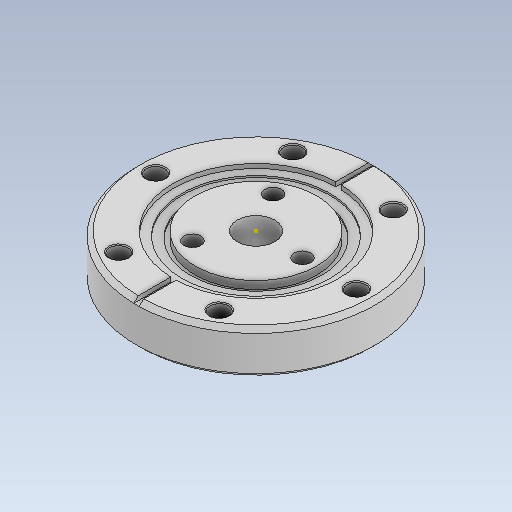
# Autodesk Inventor part: 2.75 flange
Saved by Autodesk Inventor 2020 (Build 240168000, 168)
## iProperties
Created: 2019-06-21
Part Number: 2.75 flange
Material: Generic
Document SubType Name: Modeling
Designer: ColinP
Density: 1 g/cm^3
Appearance: Default
Mass: 41.8424 g
Surface Area: 130.459 cm^2
Volume: 41.8424 cm^3
Author: ColinP
Autodesk Inventor part; units mm, degrees
ref_plane "YZ Plane" through (0, 0, 0) normal (1, 0, 0) x (0, 1, 0)
ref_plane "XZ Plane" through (0, 0, 0) normal (0, 1, 0) x (-1, 0, 0)
ref_plane "XY Plane" through (0, 0, 0) normal (0, 0, 1) x (1, 0, 0)
sketch "Sketch1" plane through (0, 0, 0) normal (0, 1, 0) x (-1, 0, 0)
  circle A0 centre (0, 0) radius 34.925
  dimension "d0" = 69.85
  constraints: 1 centre point, 1 coincident
  measures "d0" diameter of A0
extrude "Extrusion1" add sketch "Sketch1" along normal blind 12.7
sketch "Sketch2" plane through (0, 12.7, 0) normal (0, 1, 0) x (1, 0, 0)
  circle A0 centre (0, 0) radius 17.78
  circle A1 centre (0, 0) radius 19.05
  circle A2 centre (0, 0) radius 21.59
  circle A3 centre (0, 0) radius 24.13
  dimension "d3" = 35.56
  dimension "d4" = 38.1
  dimension "d5" = 43.18
  dimension "d6" = 48.26
  constraints: 4 centre point, 4 coincident
  measures "d3" diameter of A0
  measures "d4" diameter of A1
  measures "d5" diameter of A2
  measures "d6" diameter of A3
extrude "Extrusion2" cut sketch "Sketch2" against normal blind 1.27 contours A3
extrude "Extrusion3" cut sketch "Sketch2" against normal blind 1.778 contours A2
extrude "Extrusion4" cut sketch "Sketch2" against normal blind 2.286 contours A1
sketch "Sketch3" plane through (0, 0, 0) normal (0, -1, 0) x (1, 0, 0)
  circle A0 centre (0, 0) radius 19.05
  circle A1 centre (0, 0) radius 21.59
  circle A2 centre (0, 0) radius 24.13
  constraints: 3 centre point, 3 coincident
sketch "Sketch4" plane through (0, 0, 0) normal (0, -1, 0) x (1, 0, 0)
  circle A0 centre (0, 0) radius 17.78
  circle A1 centre (0, 0) radius 19.05
  constraints: 2 centre point, 2 coincident
extrude "Extrusion5" cut sketch "Sketch3" against normal blind 1.27 contours A2
extrude "Extrusion6" cut sketch "Sketch3" against normal blind 1.778 contours A1
extrude "Extrusion7" cut sketch "Sketch4" against normal blind 2.286
chamfer "Chamfer1" distance 1.27 angle 45 2 edges at (34.925, 12.7, 0) (34.925, 0, 0)
sketch "Sketch5" plane through (0, 12.7, 0) normal (0, 1, 0) x (1, 0, 0)
  point P0 (0, 0)
sketch "Sketch6" plane through (0, 12.7, 0) normal (0, 1, 0) x (1, 0, 0)
  point P0 (0, 0)
sketch "Sketch7" plane through (0, 12.7, 0) normal (0, 1, 0) x (1, 0, 0)
  line L0 (0, 0) -> (-29.3624, 0)
  dimension "d22" = 29.3624
  constraints: 2 end point, 1 horizontal
  measures "d22" distance of L0.start L0.end
hole "Hole1" at (-29.3624, 12.7, 0) direction (0, -1, 0) diameter 5.4102 end through all
chamfer "Chamfer2" distance 0.254 angle 45 1 edges at (-29.3624, 12.7, -2.7051)
chamfer "Chamfer3" distance 0.254 angle 45 1 edges at (-29.3624, 0, -2.7051)
pattern_circular "Circular Pattern1" count 6 over 360 about axis through (0, 12.7, 0) along (0, -1, 0) of "Hole1", "Chamfer2"
sketch "Sketch8" plane through (0, 12.7, 0) normal (0, 1, 0) x (1, 0, 0)
  line L0 (0, 0) -> (0.7937, 0)
  line L1 (0.7937, 0) -> (0.7937, 24.1169)
  circle A0 centre (0, 0) radius 24.13 projected
  circle A1 centre (0, 0) radius 34.925 projected
  line L2 (0.7937, 34.916) -> (0.7937, 24.1169)
  line L3 (0.7937, 0) -> (-0.7937, 0)
  line L4 (-0.7937, 0) -> (-0.7937, 34.916)
  line L5 (-0.7937, 34.916) -> (0.7937, 34.916)
  line L6 (0.7937, 5.7639) -> (0.7937, -35.1013)
  line L7 (0.7937, -35.1013) -> (-0.7937, -35.1013)
  line L8 (-0.7937, -35.1013) -> (-0.7937, 0)
  line L9 (-0.7937, -24.0567) -> (0.7937, -24.0567)
  line L10 (0.7937, 24.1169) -> (-0.7937, 24.1169)
  point P0 (-0.7937, -24.1169)
  point P1 (-0.7938, -34.916)
  point P2 (0.7937, -34.916)
  point P3 (0.7938, -24.1169)
  point P4 (-0.7937, 24.1169)
  dimension "d39" = 0.7937
  dimension "d40" = 1.5875
  constraints: 22 end point, 8 point on line, 6 perpendicular, 1 collinear, 1 horizontal, 1 parallel, 4 other
  measures "d39" distance of L0.start L0.end
  measures "d40" distance of L0.end L3.end
extrude "Extrusion8" cut sketch "Sketch8" against normal blind 1.27 contours L4 L5 L2 A0 | L6 A1 L8 A0
hole "Hole2" at (0, 12.7, 0) direction (0, -1, 0) diameter 10.9982 end through all
sketch "Sketch9" plane through (0, 12.7, 0) normal (0, 1, 0) x (1, 0, 0)
  line L0 (0, 0) -> (13.6144, 0)
  dimension "d50" = 13.6144
  constraints: 2 end point, 1 horizontal
  measures "d50" distance of L0.start L0.end
hole "Hole3" at (13.6144, 12.7, 0) direction (0, -1, 0) diameter 4.9022 end through all
pattern_circular "Circular Pattern2" count 3 over 360 about axis through (0, -86.8959, 0) along (0, 1, 0) of "Hole3"
body "Solid1"
